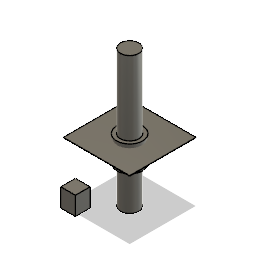
_magnetic side.8d1368b1-dcc9-4457-ae46-fbf8c22e0692 (Autodesk Fusion 360 design; units mm, degrees)
Autodesk Fusion 360 part; units mm, degrees
note: some values were not read from the file. Chosen so that the rebuilt part matches the saved one: which face or edge a step refers to.
sketch "Sketch1" plane through (0, 0, 0) normal (0, 1, 0) x (1, 0, 0)
  circle A0 centre (0, 0) radius 25
  circle A1 centre (0, 0) radius 35
  dimension "d1" = 50
  dimension "d2" = 70
  measures "d1" diameter of A0
  measures "d2" diameter of A1
extrude "Extrude1" add sketch "Sketch1" along normal blind 200 contours A0 makes body 1
extrude "Extrude2" add sketch "Sketch1" along normal blind 70 separate body contours A0 | A1 makes body 2
extrude "Extrude3" add sketch "Sketch1" along normal blind 100 separate body contours A0 makes body 3
sketch "Sketch2" plane through (0, 0, 0) normal (0, 1, 0) x (1, 0, 0)
  line L0 (20, 20) -> (-20, 20)
  line L1 (-20, 20) -> (-20, -20)
  line L2 (-20, -20) -> (20, -20)
  line L3 (20, -20) -> (20, 20)
  line L4 (20, 20) -> (-20, -20) construction
  line L5 (-20, 20) -> (20, -20) construction
  dimension "d9" = 40
  dimension "d10" = 40
  measures "d9" distance of L0.end L1.end
  measures "d10" distance of L1.end L2.end
extrude "Extrude6" add sketch "Sketch2" along normal blind 50 separate body makes body 4
copy_body "Body->Comp2" bodies 1 removing the originals makes body 5 in component "Component"
copy_body "Body->Comp3" bodies 3 removing the originals makes body 6 in component "Component'"
copy_body "Body->Comp4" bodies 2 removing the originals makes body 7 in component "Component''"
copy_body "Body->Comp5" bodies 4 removing the originals makes body 8 in component "Component'''"
sphere "SpherePrimitive1" add diameter 70 placed x (1, 0, 0) y (0, 0, -1) z (0, 1, 0) at (0, 0, 0) separate body makes body 9
copy_body "Body->Comp6" bodies 9 removing the originals makes body 10 in component "Component''''"
delete_face "DeleteFace1" 1 faces at (33.1826, -7.4475, -8.2734) on bodies 10 in component "Component''''"
sketch "Sketch4" plane through (0, 0, 0) normal (0, 1, 0) x (1, 0, 0)
  line L0 (90, 90) -> (-90, 90)
  line L1 (-90, 90) -> (-90, -90)
  line L2 (-90, -90) -> (90, -90)
  line L3 (90, -90) -> (90, 90)
  line L4 (90, 90) -> (-90, -90) construction
  line L5 (-90, 90) -> (90, -90) construction
  dimension "d18" = 180
  dimension "d19" = 180
  measures "d18" distance of L1.end L2.end
  measures "d19" distance of L0.end L1.end
extrude "Extrude7" add sketch "Sketch4" along normal blind 1 separate body makes body 11
copy_body "Body->Comp7" bodies 11 removing the originals makes body 12 in component "Component'''''"
move_body "Move1" bodies 12 to x (1, 0, 0) y (0, 1, 0) z (0, 0, 1) at (0, 160, 0) in component "Component'''''"
component "Component" placed x (1, 0, 0) y (0, 1, 0) z (0, 0, 1) at (0, 170, 0)
component "Component'" placed x (1, 0, 0) y (0, 1, 0) z (0, 0, 1) at (0, 0, 0)
component "Component''" placed x (1, 0, 0) y (0, 1, 0) z (0, 0, 1) at (0, 100, 0)
component "Component'''" placed x (1, 0, 0) y (0, 1, 0) z (0, 0, 1) at (-68.0379, -1.0122, 148.0032)
component "Component''''" placed x (1, 0, 0) y (0, 1, 0) z (0, 0, 1) at (0, 290, 0)
component "Component'''''" placed x (1, 0, 0) y (0, 1, 0) z (0, 0, 1) at (0, 0, 0)
